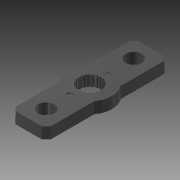
# Autodesk Inventor part: Shaft Lock Bar
Saved by Autodesk Inventor 2013 (Build 170138000, 138)
## iProperties
Created: 2010-06-22
Part Number: Shaft Lock Bar
Document SubType Name: Modeling
Designer: Phil
Density: 1 g/cm^3
Material: Generic
Author: Phil
Autodesk Inventor part; units mm, degrees
ref_plane "YZ Plane" through (0, 0, 0) normal (1, 0, 0) x (0, 1, 0)
ref_plane "XZ Plane" through (0, 0, 0) normal (0, 1, 0) x (-1, 0, 0)
ref_plane "XY Plane" through (0, 0, 0) normal (0, 0, 1) x (1, 0, 0)
sketch "Sketch1" plane through (0, 0, 0) normal (0, 0, 1) x (1, 0, 0)
  arc A0 (20.278526, 10.04916) -> (12.695563, 10.04916) centre (16.487044, 5.02458) ccw
  line L0 (12.695563, 10.04916) -> (0, 10.04916)
  line L1 (0, 10.04916) -> (-1.237536, 8.811625)
  line L2 (-1.237536, 8.811625) -> (-1.237536, 1.237536)
  line L3 (-1.237536, 1.237536) -> (0, 0)
  line L4 (0, 0) -> (12.695563, 0)
  arc A1 (12.695563, 0) -> (20.278526, 0) centre (16.487044, 5.02458) ccw
  line L5 (20.278526, 0) -> (32.974089, 0)
  line L6 (32.974089, 0) -> (34.211625, 1.237536)
  line L7 (34.211625, 1.237536) -> (34.211625, 8.811625)
  line L8 (34.211625, 8.811625) -> (32.974089, 10.04916)
  line L9 (32.974089, 10.04916) -> (20.278526, 10.04916)
  arc A2 (15.472273, 7.960642) -> (15.128487, 7.818241) centre (16.487044, 5.02458) ccw
  arc A3 (15.897832, 8.07467) -> (15.472273, 7.960642) centre (15.675155, 8.054593) ccw
  arc A4 (16.267312, 8.123279) -> (15.897832, 8.07467) centre (16.487044, 5.02458) ccw
  arc A5 (16.706777, 8.123279) -> (16.267312, 8.123279) centre (16.487044, 8.16458) ccw
  arc A6 (17.076802, 8.074565) -> (16.706777, 8.123279) centre (16.487044, 5.02458) ccw
  arc A7 (17.501292, 7.960823) -> (17.076802, 8.074565) centre (17.299736, 8.057587) ccw
  arc A8 (17.8461, 7.817999) -> (17.501292, 7.960823) centre (16.487044, 5.02458) ccw
  arc A9 (18.226688, 7.598266) -> (17.8461, 7.817999) centre (18.057044, 7.7439) ccw
  arc A10 (18.522781, 7.371066) -> (18.226688, 7.598266) centre (16.487044, 5.02458) ccw
  arc A11 (18.83353, 7.060317) -> (18.522781, 7.371066) centre (18.70736, 7.244895) ccw
  arc A12 (19.06073, 6.764224) -> (18.83353, 7.060317) centre (16.487044, 5.02458) ccw
  arc A13 (19.280463, 6.383636) -> (19.06073, 6.764224) centre (19.206364, 6.59458) ccw
  arc A14 (19.423287, 6.038828) -> (19.280463, 6.383636) centre (16.487044, 5.02458) ccw
  arc A15 (19.537029, 5.614337) -> (19.423287, 6.038828) centre (19.520051, 5.837272) ccw
  arc A16 (19.585744, 5.244313) -> (19.537029, 5.614337) centre (16.487044, 5.02458) ccw
  arc A17 (19.585744, 4.804848) -> (19.585744, 5.244313) centre (19.627044, 5.02458) ccw
  arc A18 (19.537029, 4.434823) -> (19.585744, 4.804848) centre (16.487044, 5.02458) ccw
  arc A19 (19.423287, 4.010333) -> (19.537029, 4.434823) centre (19.520051, 4.211888) ccw
  arc A20 (19.280463, 3.665524) -> (19.423287, 4.010333) centre (16.487044, 5.02458) ccw
  arc A21 (19.06073, 3.284937) -> (19.280463, 3.665524) centre (19.206364, 3.45458) ccw
  arc A22 (18.83353, 2.988843) -> (19.06073, 3.284937) centre (16.487044, 5.02458) ccw
  arc A23 (18.522781, 2.678095) -> (18.83353, 2.988843) centre (18.70736, 2.804265) ccw
  arc A24 (18.226688, 2.450894) -> (18.522781, 2.678095) centre (16.487044, 5.02458) ccw
  arc A25 (17.8461, 2.231162) -> (18.226688, 2.450894) centre (18.057044, 2.30526) ccw
  arc A26 (17.501292, 2.088338) -> (17.8461, 2.231162) centre (16.487044, 5.02458) ccw
  arc A27 (17.076802, 1.974596) -> (17.501292, 2.088338) centre (17.299736, 1.991573) ccw
  arc A28 (16.706777, 1.925881) -> (17.076802, 1.974596) centre (16.487044, 5.02458) ccw
  arc A29 (16.267312, 1.925881) -> (16.706777, 1.925881) centre (16.487044, 1.88458) ccw
  arc A30 (15.897287, 1.974596) -> (16.267312, 1.925881) centre (16.487044, 5.02458) ccw
  arc A31 (15.472797, 2.088338) -> (15.897287, 1.974596) centre (15.674353, 1.991573) ccw
  arc A32 (15.127989, 2.231162) -> (15.472797, 2.088338) centre (16.487044, 5.02458) ccw
  arc A33 (14.747401, 2.450894) -> (15.127989, 2.231162) centre (14.917044, 2.30526) ccw
  arc A34 (14.451307, 2.678095) -> (14.747401, 2.450894) centre (16.487044, 5.02458) ccw
  arc A35 (14.140559, 2.988843) -> (14.451307, 2.678095) centre (14.266729, 2.804265) ccw
  arc A36 (13.913358, 3.284937) -> (14.140559, 2.988843) centre (16.487044, 5.02458) ccw
  arc A37 (13.693626, 3.665524) -> (13.913358, 3.284937) centre (13.767725, 3.45458) ccw
  arc A38 (13.550802, 4.010333) -> (13.693626, 3.665524) centre (16.487044, 5.02458) ccw
  arc A39 (13.43706, 4.434823) -> (13.550802, 4.010333) centre (13.454037, 4.211888) ccw
  arc A40 (13.388384, 4.804294) -> (13.43706, 4.434823) centre (16.487044, 5.02458) ccw
  arc A41 (13.388384, 5.244866) -> (13.388384, 4.804294) centre (13.350144, 5.02458) ccw
  arc A42 (13.436955, 5.613793) -> (13.388384, 5.244866) centre (16.487044, 5.02458) ccw
  arc A43 (13.550983, 6.039352) -> (13.436955, 5.613793) centre (13.457032, 5.83647) ccw
  arc A44 (13.693383, 6.383137) -> (13.550983, 6.039352) centre (16.487044, 5.02458) ccw
  arc A45 (13.913669, 6.764683) -> (13.693383, 6.383137) centre (13.770409, 6.59303) ccw
  arc A46 (14.140195, 7.059898) -> (13.913669, 6.764683) centre (16.487044, 5.02458) ccw
  arc A47 (14.451726, 7.371429) -> (14.140195, 7.059898) centre (14.268921, 7.242703) ccw
  arc A48 (14.746941, 7.597956) -> (14.451726, 7.371429) centre (16.487044, 5.02458) ccw
  arc A49 (15.128487, 7.818241) -> (14.746941, 7.597956) centre (14.918594, 7.741215) ccw
  line L10 (21.973444, 4.14828) -> (20.449444, 5.02458)
  line L11 (20.449444, 5.02458) -> (21.973444, 5.90088)
  line L12 (21.973444, 5.90088) -> (21.973444, 4.14828)
  circle A50 centre (3.787044, 5.02458) radius 2.3114
  circle A51 centre (29.187044, 5.02458) radius 2.3114
  circle A52 centre (10.598444, 5.02458) radius 1
  point P0 (0, 0)
  constraints: 100 point on circle, 53 centre point, 26 end point
sketch "Sketch1 outline for Extrusion1" plane through (0, 0, 0) normal (0, 0, 1) x (1, 0, 0)
  line L0 (12.695563, 0) -> (0, 0)
  line L1 (0, 0) -> (-1.237536, 1.237536)
  line L2 (-1.237536, 1.237536) -> (-1.237536, 8.811625)
  line L3 (-1.237536, 8.811625) -> (0, 10.04916)
  line L4 (0, 10.04916) -> (12.695563, 10.04916)
  arc A0 (12.695563, 10.04916) -> (20.278526, 10.04916) centre (16.487044, 5.02458) cw
  line L5 (20.278526, 10.04916) -> (32.974089, 10.04916)
  line L6 (32.974089, 10.04916) -> (34.211625, 8.811625)
  line L7 (34.211625, 8.811625) -> (34.211625, 1.237536)
  line L8 (34.211625, 1.237536) -> (32.974089, 0)
  line L9 (32.974089, 0) -> (20.278526, 0)
  arc A1 (20.278526, 0) -> (12.695563, 0) centre (16.487044, 5.02458) cw
extrude "Extrusion1" add sketch "Sketch1 outline for Extrusion1" along normal blind 3.175 draft 2
hole "Hole1" at (3.787044, 5.02458, 0) at (29.187044, 5.02458, 0) direction (0, 0, 1) diameter 4.6228 end up to surface
extrude "Extrusion2" cut sketch "Sketch1" along normal blind 0.254 contours L10 L11 L12 | A52
extrude "Extrusion3" cut sketch "Sketch1" along normal up to next draft 2 contours A3 A4 A5 A6 A7 A8 A9 A10 A11 A12 A13 A14 A15 A16 A17 A18 A19 A20 A21 A22 A23 A24 A25 A26 A27 A28 A29 A30 A31 A32 A33 A34 A35 A36 A37 A38 A39 A40 A41 A42 A43 A44 A45 A46 A47 A48 A49 A2
sketch "Sketch2" plane through (0, 0, 3.175) normal (0, 0, 1) x (1, 0, 0)
  line L0 (-1.292956, 1.21458) -> (-1.292956, 8.83458)
  line L1 (-0.022956, -0.05542) -> (-1.292956, 1.21458)
  line L2 (12.677044, -0.05542) -> (-0.022956, -0.05542)
  arc A0 (12.677044, -0.05542) -> (20.297044, -0.05542) centre (16.487044, 5.02458) ccw
  line L3 (32.997044, -0.05542) -> (20.297044, -0.05542)
  line L4 (34.267044, 1.21458) -> (32.997044, -0.05542)
  line L5 (34.267044, 8.83458) -> (34.267044, 1.21458)
  line L6 (32.997044, 10.10458) -> (34.267044, 8.83458)
  line L7 (20.297044, 10.10458) -> (32.997044, 10.10458)
  arc A1 (20.297044, 10.10458) -> (12.677044, 10.10458) centre (16.487044, 5.02458) ccw
  line L8 (-0.022956, 10.10458) -> (12.677044, 10.10458)
  line L9 (-1.292956, 8.83458) -> (-0.022956, 10.10458)
  ellipse E0 centre (2.786968, 1.444599) end of major axis (3.234274, 1.220963) minor radius 0.5 (2.787044, 0.94458) -> (3.284648, 1.395632) ccw
  line L10 (0.598357, 0.94458) -> (2.787044, 0.94458)
  arc A2 (0.244817, 1.091021) -> (0.598357, 0.94458) centre (0.598356, 1.44456) ccw
  line L11 (0.244817, 1.091021) -> (-0.146515, 1.482353)
  arc A3 (-0.292956, 1.835893) -> (-0.146515, 1.482353) centre (0.207024, 1.835892) ccw
  line L12 (-0.292956, 4.02458) -> (-0.292956, 1.835893)
  ellipse E1 centre (0.207063, 4.024504) end of major axis (0.430699, 3.577198) minor radius 0.5 (0.158097, 4.522184) -> (-0.292956, 4.02458) ccw
  spline S0 degree 3 poles (0.158097, 4.522184) (0.207081, 4.517371) (0.255087, 4.505349) (0.348213, 4.466766) (0.392524, 4.439766) (0.471313, 4.373174) (0.505317, 4.333983) (0.558882, 4.248592) (0.578739, 4.203259) (0.591653, 4.155761) knots 0 0 0 0 0.24414505 0.24414505 0.5000027 0.5000027 0.75584477 0.75584477 1 1 1 1
  arc A4 (0.591653, 4.155761) -> (2.918225, 1.829189) centre (3.787044, 5.02458) ccw
  spline S1 degree 3 poles (2.918225, 1.829189) (2.965724, 1.816275) (3.011056, 1.796418) (3.096447, 1.742853) (3.135638, 1.708849) (3.20223, 1.63006) (3.22923, 1.585748) (3.267813, 1.492623) (3.279835, 1.444617) (3.284648, 1.395632) knots 0 0 0 0 0.24415523 0.24415523 0.4999973 0.4999973 0.75585495 0.75585495 1 1 1 1
  ellipse E2 centre (32.767025, 4.024504) end of major axis (32.990661, 4.47181) minor radius 0.5 (33.267044, 4.02458) -> (32.815992, 4.522184) ccw
  line L13 (33.267044, 1.835893) -> (33.267044, 4.02458)
  arc A5 (33.120603, 1.482353) -> (33.267044, 1.835893) centre (32.767065, 1.835892) ccw
  line L14 (33.120603, 1.482353) -> (32.729272, 1.091021)
  arc A6 (32.375732, 0.94458) -> (32.729272, 1.091021) centre (32.375733, 1.44456) ccw
  line L15 (30.187044, 0.94458) -> (32.375732, 0.94458)
  ellipse E3 centre (30.187121, 1.444599) end of major axis (29.739815, 1.220963) minor radius 0.5 (29.689441, 1.395632) -> (30.187044, 0.94458) ccw
  spline S2 degree 3 poles (29.689441, 1.395632) (29.694254, 1.444617) (29.706275, 1.492623) (29.744859, 1.585748) (29.771859, 1.63006) (29.83845, 1.708849) (29.877641, 1.742853) (29.963033, 1.796418) (30.008365, 1.816275) (30.055863, 1.829189) knots 0 0 0 0 0.24414505 0.24414505 0.5000027 0.5000027 0.75584477 0.75584477 1 1 1 1
  arc A7 (30.055863, 1.829189) -> (32.382435, 4.155761) centre (29.187044, 5.02458) ccw
  spline S3 degree 3 poles (32.382435, 4.155761) (32.39535, 4.203259) (32.415207, 4.248592) (32.468771, 4.333983) (32.502776, 4.373174) (32.581564, 4.439766) (32.625876, 4.466766) (32.719002, 4.505349) (32.767008, 4.517371) (32.815992, 4.522184) knots 0 0 0 0 0.24415523 0.24415523 0.4999973 0.4999973 0.75585495 0.75585495 1 1 1 1
  line L16 (32.729272, 8.958139) -> (33.120603, 8.566808)
  arc A8 (33.267044, 8.213268) -> (33.120603, 8.566808) centre (32.767065, 8.213268) ccw
  line L17 (33.267044, 6.02458) -> (33.267044, 8.213268)
  ellipse E4 centre (32.767025, 6.024656) end of major axis (32.990661, 5.577351) minor radius 0.5 (32.815992, 5.526976) -> (33.267044, 6.02458) ccw
  spline S4 degree 3 poles (32.815992, 5.526976) (32.767008, 5.53179) (32.719002, 5.543811) (32.625876, 5.582394) (32.581564, 5.609395) (32.502776, 5.675986) (32.468771, 5.715177) (32.415207, 5.800569) (32.39535, 5.845901) (32.382435, 5.893399) knots 0 0 0 0 0.24414505 0.24414505 0.5000027 0.5000027 0.75584477 0.75584477 1 1 1 1
  arc A9 (32.382435, 5.893399) -> (30.055863, 8.219971) centre (29.187044, 5.02458) ccw
  spline S5 degree 3 poles (30.055863, 8.219971) (30.008365, 8.232886) (29.963033, 8.252742) (29.877641, 8.306307) (29.83845, 8.340312) (29.771859, 8.4191) (29.744859, 8.463412) (29.706275, 8.556538) (29.694254, 8.604544) (29.689441, 8.653528) knots 0 0 0 0 0.24415523 0.24415523 0.4999973 0.4999973 0.75585495 0.75585495 1 1 1 1
  ellipse E5 centre (30.187121, 8.604561) end of major axis (30.634426, 8.380925) minor radius 0.5 (30.187044, 9.10458) -> (29.689441, 8.653528) ccw
  line L18 (32.375732, 9.10458) -> (30.187044, 9.10458)
  arc A10 (32.729272, 8.958139) -> (32.375732, 9.10458) centre (32.375733, 8.604601) ccw
  arc A11 (6.989234, 5.867997) -> (4.655863, 8.219971) centre (3.787044, 5.02458) ccw
  spline S6 degree 3 poles (4.655863, 8.219971) (4.608365, 8.232886) (4.563033, 8.252742) (4.477641, 8.306307) (4.43845, 8.340311) (4.371859, 8.4191) (4.344858, 8.463412) (4.306275, 8.556537) (4.294254, 8.604543) (4.289441, 8.653528) knots 0 0 0 0 0.24415523 0.24415523 0.4999973 0.4999973 0.75585495 0.75585495 1 1 1 1
  ellipse E6 centre (4.787121, 8.604561) end of major axis (5.234426, 8.380925) minor radius 0.5 (4.787044, 9.10458) -> (4.289441, 8.653528) ccw
  line L19 (11.747265, 9.10458) -> (4.787044, 9.10458)
  arc A12 (11.981811, 8.617529) -> (11.747265, 9.10458) centre (11.747265, 8.80458) ccw
  arc A13 (11.981811, 8.617529) -> (10.794199, 5.91784) centre (16.487044, 5.02458) ccw
  spline S7 degree 3 poles (10.794199, 5.91784) (10.785332, 5.861333) (10.766837, 5.806763) (10.710367, 5.702889) (10.671644, 5.655056) (10.578884, 5.575704) (10.525627, 5.544854) (10.414258, 5.505158) (10.357484, 5.495343) (10.300288, 5.495343) knots 0 0 0 0 0.24188929 0.24188929 0.49999623 0.49999623 0.75811855 0.75811855 1 1 1 1
  line L20 (7.472706, 5.495343) -> (10.300288, 5.495343)
  spline S8 degree 3 poles (7.472706, 5.495343) (7.419393, 5.495343) (7.366421, 5.503871) (7.262283, 5.538295) (7.212141, 5.56491) (7.122857, 5.633733) (7.084355, 5.675445) (7.024551, 5.767385) (7.002813, 5.81644) (6.989234, 5.867997) knots 0 0 0 0 0.24304225 0.24304225 0.50000313 0.50000313 0.75694938 0.75694938 1 1 1 1
  line L21 (4.787044, 0.94458) -> (11.747265, 0.94458)
  ellipse E7 centre (4.787121, 1.444599) end of major axis (4.339815, 1.220963) minor radius 0.5 (4.289441, 1.395632) -> (4.787044, 0.94458) ccw
  spline S9 degree 3 poles (4.289441, 1.395632) (4.294254, 1.444617) (4.306275, 1.492623) (4.344859, 1.585748) (4.371859, 1.63006) (4.43845, 1.708849) (4.477641, 1.742853) (4.563033, 1.796418) (4.608365, 1.816275) (4.655863, 1.829189) knots 0 0 0 0 0.24414505 0.24414505 0.5000027 0.5000027 0.75584477 0.75584477 1 1 1 1
  arc A14 (4.655863, 1.829189) -> (6.989234, 4.181163) centre (3.787044, 5.02458) ccw
  spline S10 degree 3 poles (6.989234, 4.181163) (7.002813, 4.23272) (7.02455, 4.281776) (7.084355, 4.373715) (7.122857, 4.415428) (7.21214, 4.48425) (7.262283, 4.510866) (7.366421, 4.54529) (7.419392, 4.553818) (7.472706, 4.553817) knots 0 0 0 0 0.24305062 0.24305062 0.49999687 0.49999687 0.75695775 0.75695775 1 1 1 1
  line L22 (10.300288, 4.553817) -> (7.472706, 4.553817)
  spline S11 degree 3 poles (10.300288, 4.553817) (10.357484, 4.553817) (10.414258, 4.544002) (10.525627, 4.504306) (10.578884, 4.473457) (10.671644, 4.394105) (10.710367, 4.346271) (10.766837, 4.242397) (10.785332, 4.187828) (10.794199, 4.131321) knots 0 0 0 0 0.24188145 0.24188145 0.50000377 0.50000377 0.75811071 0.75811071 1 1 1 1
  arc A15 (10.794199, 4.131321) -> (11.981811, 1.431632) centre (16.487044, 5.02458) ccw
  arc A16 (11.747265, 0.94458) -> (11.981811, 1.431632) centre (11.747265, 1.24458) ccw
  arc A17 (25.984855, 4.181163) -> (28.318225, 1.829189) centre (29.187044, 5.02458) ccw
  spline S12 degree 3 poles (28.318225, 1.829189) (28.365724, 1.816275) (28.411056, 1.796418) (28.496447, 1.742853) (28.535638, 1.708849) (28.60223, 1.63006) (28.62923, 1.585748) (28.667813, 1.492623) (28.679835, 1.444617) (28.684648, 1.395632) knots 0 0 0 0 0.24415523 0.24415523 0.4999973 0.4999973 0.75585495 0.75585495 1 1 1 1
  ellipse E8 centre (28.186968, 1.444599) end of major axis (28.634274, 1.220963) minor radius 0.5 (28.187044, 0.94458) -> (28.684648, 1.395632) ccw
  line L23 (21.226823, 0.94458) -> (28.187044, 0.94458)
  arc A18 (20.992278, 1.431632) -> (21.226823, 0.94458) centre (21.226823, 1.24458) ccw
  arc A19 (20.992278, 1.431632) -> (22.17989, 4.131321) centre (16.487044, 5.02458) ccw
  spline S13 degree 3 poles (22.17989, 4.131321) (22.188757, 4.187828) (22.207252, 4.242397) (22.263722, 4.346271) (22.302445, 4.394105) (22.395204, 4.473457) (22.448461, 4.504306) (22.559831, 4.544002) (22.616605, 4.553817) (22.673801, 4.553817) knots 0 0 0 0 0.24188929 0.24188929 0.49999623 0.49999623 0.75811855 0.75811855 1 1 1 1
  line L24 (25.501383, 4.553817) -> (22.673801, 4.553817)
  spline S14 degree 3 poles (25.501383, 4.553817) (25.554696, 4.553817) (25.607668, 4.545289) (25.711805, 4.510865) (25.761948, 4.48425) (25.851232, 4.415428) (25.889734, 4.373715) (25.949538, 4.281776) (25.971275, 4.23272) (25.984855, 4.181163) knots 0 0 0 0 0.24304225 0.24304225 0.50000313 0.50000313 0.75694938 0.75694938 1 1 1 1
  arc A20 (22.17989, 5.91784) -> (20.992278, 8.617529) centre (16.487044, 5.02458) ccw
  arc A21 (21.226823, 9.10458) -> (20.992278, 8.617529) centre (21.226823, 8.80458) ccw
  line L25 (28.187044, 9.10458) -> (21.226823, 9.10458)
  ellipse E9 centre (28.186968, 8.604561) end of major axis (27.739663, 8.380925) minor radius 0.5 (28.684648, 8.653528) -> (28.187044, 9.10458) ccw
  spline S15 degree 3 poles (28.684648, 8.653528) (28.679835, 8.604544) (28.667813, 8.556538) (28.62923, 8.463412) (28.60223, 8.4191) (28.535638, 8.340312) (28.496447, 8.306307) (28.411056, 8.252742) (28.365724, 8.232886) (28.318225, 8.219971) knots 0 0 0 0 0.24414505 0.24414505 0.5000027 0.5000027 0.75584477 0.75584477 1 1 1 1
  arc A22 (28.318225, 8.219971) -> (25.984855, 5.867997) centre (29.187044, 5.02458) ccw
  spline S16 degree 3 poles (25.984855, 5.867997) (25.971275, 5.81644) (25.949538, 5.767385) (25.889734, 5.675445) (25.851232, 5.633733) (25.761948, 5.56491) (25.711806, 5.538295) (25.607668, 5.503871) (25.554696, 5.495343) (25.501383, 5.495343) knots 0 0 0 0 0.24305062 0.24305062 0.49999687 0.49999687 0.75695775 0.75695775 1 1 1 1
  line L26 (22.673801, 5.495343) -> (25.501383, 5.495343)
  spline S17 degree 3 poles (22.673801, 5.495343) (22.616605, 5.495343) (22.559831, 5.505158) (22.448461, 5.544854) (22.395204, 5.575704) (22.302445, 5.655056) (22.263722, 5.702889) (22.207252, 5.806763) (22.188757, 5.861333) (22.17989, 5.91784) knots 0 0 0 0 0.24188145 0.24188145 0.50000377 0.50000377 0.75811071 0.75811071 1 1 1 1
  circle A23 centre (16.487044, 5.02458) radius 4.7625
  circle A24 centre (29.187044, 5.02458) radius 2.36682
  circle A25 centre (3.787044, 5.02458) radius 2.36682
  line L27 (-0.146515, 8.566808) -> (0.244817, 8.958139)
  arc A26 (0.598357, 9.10458) -> (0.244817, 8.958139) centre (0.598356, 8.604601) ccw
  line L28 (2.787044, 9.10458) -> (0.598357, 9.10458)
  ellipse E10 centre (2.786968, 8.604561) end of major axis (2.339663, 8.380925) minor radius 0.5 (3.284648, 8.653528) -> (2.787044, 9.10458) ccw
  spline S18 degree 3 poles (3.284648, 8.653528) (3.279835, 8.604544) (3.267813, 8.556538) (3.22923, 8.463412) (3.20223, 8.4191) (3.135638, 8.340312) (3.096447, 8.306307) (3.011056, 8.252742) (2.965724, 8.232886) (2.918225, 8.219971) knots 0 0 0 0 0.24414505 0.24414505 0.5000027 0.5000027 0.75584477 0.75584477 1 1 1 1
  arc A27 (2.918225, 8.219971) -> (0.591653, 5.893399) centre (3.787044, 5.02458) ccw
  spline S19 degree 3 poles (0.591653, 5.893399) (0.578739, 5.845901) (0.558882, 5.800569) (0.505317, 5.715177) (0.471313, 5.675986) (0.392524, 5.609395) (0.348213, 5.582394) (0.255087, 5.543811) (0.207081, 5.53179) (0.158097, 5.526976) knots 0 0 0 0 0.24415523 0.24415523 0.4999973 0.4999973 0.75585495 0.75585495 1 1 1 1
  ellipse E11 centre (0.207063, 6.024656) end of major axis (0.430699, 6.471962) minor radius 0.5 (-0.292956, 6.02458) -> (0.158097, 5.526976) ccw
  line L29 (-0.292956, 8.213268) -> (-0.292956, 6.02458)
  arc A28 (-0.146515, 8.566808) -> (-0.292956, 8.213268) centre (0.207024, 8.213268) ccw
  point P0 (0, 0)
  constraints: 60 end point, 52 point on circle, 29 centre point, 88 other
extrude "Extrusion4" cut sketch "Sketch2" against normal blind 1.6764 contours L10 A2 L11 A3 L12 E1 S0 A4 S1 E0 | L13 A5 L14 A6 L15 E3 S2 A7 S3 E2 | L16 A8 L17 E4 S4 A9 S5 E5 L18 A10 | A11 S6 E6 L19 A12 A13 S7 L20 S8 | E7 S9 A14 S10 L22 S11 A15 A16 L21 | A17 S12 E8 L23 A18 A19 S13 L24 S14 | A20 A21 L25 E9 S15 A22 S16 L26 S17 | L27 A26 L28 E10 S18 A27 S19 E11 L29 A28
body "Solid1"
